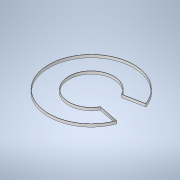
# Autodesk Inventor part: Level 1 Edge Banding
Saved by Autodesk Inventor 2020 (Build 240168000, 168)
## iProperties
Created: 2020-07-30
Part Number: Level 1 Edge Banding
Material: Generic
Document SubType Name: Modeling
Designer: Dan Wikman
Density: 1 g/cm^3
Appearance: Default
Author: Dan Wikman
Autodesk Inventor part; units mm, degrees
ref_plane "YZ Plane" through (0, 0, 0) normal (1, 0, 0) x (0, 1, 0)
ref_plane "XZ Plane" through (0, 0, 0) normal (0, 1, 0) x (-1, 0, 0)
ref_plane "XY Plane" through (0, 0, 0) normal (0, 0, 1) x (1, 0, 0)
sketch "Sketch1" plane through (0, 0, 0) normal (0, 1, 0) x (-1, 0, 0)
  arc A0 (472.3938, 0) -> (145.9777, 449.2732) centre (0, 0) ccw
  arc A1 (77.994, -240.0408) -> (252.3938, 0) centre (0, 0) ccw
  line L0 (-442.5303, 165.2961) -> (-220.837, 122.2033)
  line L1 (-442.5303, -165.2961) -> (-220.837, -122.2033)
  arc A2 (252.3938, 0) -> (-220.837, 122.2033) centre (0, 0) ccw
  arc A3 (-220.837, -122.2033) -> (77.994, -240.0408) centre (0, 0) ccw
  arc A4 (145.9777, 449.2732) -> (-442.5303, 165.2961) centre (0, 0) ccw
  arc A5 (-442.5303, -165.2961) -> (472.3938, 0) centre (0, 0) ccw
  arc A6 (-218.7278, -117.7184) -> (-218.7278, 117.7184) centre (0, 0) ccw
  arc A7 (-447.907, -162.2663) -> (-447.907, 162.2663) centre (0, 0) ccw
  line L2 (-218.7278, 117.7184) -> (-447.907, 162.2663)
  line L3 (-218.7278, -117.7184) -> (-447.907, -162.2663)
  dimension "d41" = 4
  dimension "d42" = 4
  dimension "d43" = 4
  dimension "d44" = 4
  constraints: 16 point on circle, 8 centre point, 8 end point, 4 coincident, 2 parallel, 3 other
  measures "d41" radial gap between concentric circles of A6 A2
  measures "d42" radial gap between concentric circles of A7 A4
  measures "d43" distance between parallel lines of L0 L2
  measures "d44" distance between parallel lines of L1 L3
extrude "Extrusion1" add sketch "Sketch1" along normal blind 30
body "Solid1"
